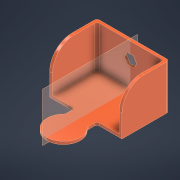
# Autodesk Inventor part: Prototype Base
Saved by Autodesk Inventor 2022 (Build 260153000, 153)
## iProperties
Created: 2021-05-30
Part Number: Prototype Base
Material: Generic
Document SubType Name: Modeling
Designer: sidsa
Density: 1 g/cm^3
Appearance: Smooth - Light Orange
Author: sidsa
## iProperties of the stored document Prototype Base_3DPrint.ipt
Created: 2021-05-30
Part Number: Prototype Base_3DPrint
Material: Generic
Document SubType Name: Modeling
Designer: sidsa
Density: 1 g/cm^3
Appearance: Default
Author: sidsa
Autodesk Inventor part; units mm, degrees
ref_plane "YZ Plane" through (0, 0, 0) normal (1, 0, 0) x (0, 1, 0)
ref_plane "XZ Plane" through (0, 0, 0) normal (0, 1, 0) x (-1, 0, 0)
ref_plane "XY Plane" through (0, 0, 0) normal (0, 0, 1) x (1, 0, 0)
sketch "Sketch1" plane through (0, 0, 0) normal (0, 1, 0) x (-1, 0, 0)
  line L0 (0, 0) -> (76.2, 0)
  line L1 (76.2, 0) -> (76.2, -50.8)
  line L2 (76.2, -50.8) -> (0, -50.8)
  line L3 (0, -50.8) -> (0, 0)
  line L4 (50.8, 0) -> (25.4, 0)
  line L5 (25.4, 0) -> (25.4, 25.4)
  line L6 (25.4, 25.4) -> (50.8, 25.4)
  line L7 (50.8, 25.4) -> (50.8, 0)
  circle A0 centre (38.1, 25.4) radius 19.05
  point P0 (52.299, 0)
  point P1 (23.901, 0)
  point P2 (50.8, 11.201)
  point P3 (25.4, 11.201)
  dimension "d0" = 76.2
  dimension "d1" = 50.8
  dimension "d2" = 25.4
  dimension "d3" = 25.4
  dimension "d4" = 25.4
  dimension "d5" = 38.1
  constraints: 16 end point, 4 parallel, 2 horizontal, 2 perpendicular, 1 centre point, 1 midpoint, 1 point on line
  measures "d0" distance of L1.end L2.end
  measures "d1" distance of L0.end L1.end
  measures "d2" distance of L5.end L6.end
  measures "d3" distance between parallel lines of L1 L7
  measures "d4" distance of L6.end L4.start
  measures "d5" diameter of A0
extrude "Extrusion2" add sketch "Sketch1" along normal blind 3.175
fillet "Fillet2" radius 3.175 4 edges at (-50.8, 1.5875, 11.201) (-50.8, 1.5875, 0) (-25.4, 1.5875, 0) (-25.4, 1.5875, 11.201)
sketch "Sketch2" plane through (0, 0, 0) normal (0, -1, 0) x (1, 0, 0)
  line L0 (0, 0) -> (0, -50.8) projected
  line L1 (0, 0) -> (3.175, 0)
  line L2 (3.175, 0) -> (3.175, -50.8)
  line L3 (3.175, -50.8) -> (0, -50.8)
  line L4 (0, -50.8) -> (0, 0)
  line L5 (-76.2, -50.8) -> (-76.2, 0) projected
  line L6 (-76.2, -50.8) -> (-79.375, -50.8)
  line L7 (-79.375, -50.8) -> (-79.375, 0)
  line L8 (-79.375, 0) -> (-76.2, 0)
  line L9 (-76.2, 0) -> (-76.2, -50.8)
  line L10 (3.175, -50.8) -> (-79.375, -50.8)
  line L11 (-79.375, -50.8) -> (-79.375, -53.975)
  line L12 (-79.375, -53.975) -> (3.175, -53.975)
  line L13 (3.175, -53.975) -> (3.175, -50.8)
  dimension "d12" = 3.175
  dimension "d13" = 3.175
  dimension "d14" = 3.175
  constraints: 24 end point, 6 parallel, 3 horizontal, 3 perpendicular, 1 point on line
  measures "d12" distance of L2.end L3.end
  measures "d13" distance of L5.start L6.end
  measures "d14" distance of L10.end L11.end
extrude "Extrusion3" add sketch "Sketch2" against normal blind 50.8
fillet "Fillet3" radius 3.175 4 edges at (3.175, 25.4, -53.975) (-79.375, 25.4, -53.975) (-76.2, 26.9875, -50.8) (0, 26.9875, -50.8)
fillet "Fillet4" radius 25.4 2 edges at (1.5875, 50.8, 0) (-77.7875, 50.8, 0)
ref_plane "Work Plane1" through (-38.1, 0, 0) normal (1, 0, 0) x (0, 0, -1)
sketch "Sketch5" plane through (0, 0, -53.975) normal (0, 0, -1) x (-1, 0, 0)
  line L0 (76.2, 50.8) -> (76.2, 0) projected
  line L1 (0, 50.8) -> (76.2, 50.8) projected
  line L2 (0, 0) -> (0, 50.8) projected
  line L3 (76.2, 0) -> (0, 0) projected
  line L4 (34.3039, 38.1) -> (41.6363, 38.1)
  line L5 (41.6363, 38.1) -> (45.3025, 31.75)
  line L6 (45.3025, 31.75) -> (41.6363, 25.4)
  line L7 (41.6363, 25.4) -> (34.3039, 25.4)
  line L8 (34.3039, 25.4) -> (30.6378, 31.75)
  line L9 (30.6378, 31.75) -> (34.3039, 38.1)
  line L10 (0, 50.8) -> (76.2, 50.8) projected
  point P0 (0, 0)
  point P1 (37.9701, 31.75)
  dimension "d27" = 12.7
  dimension "d28" = 12.7
  constraints: 12 end point, 1 parallel, 13 other
  measures "d27" distance between parallel lines of L7 L4
  measures "d28" distance between parallel lines of L1 L4
extrude "Extrusion6" cut sketch "Sketch5" against normal blind 25.4 contours L4 L5 L6 L7 L8 L9
body "Solid2"
